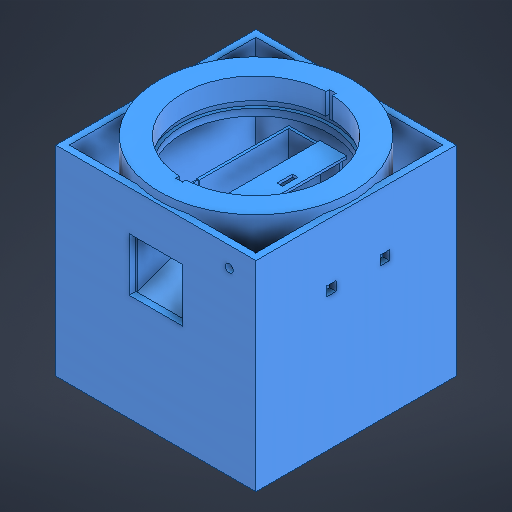
# Autodesk Inventor part: Box na elektrotechniku oprava
Saved by Autodesk Inventor 2026.2 (Build 302298000, 298)
## iProperties
Created: 2025-09-11
Part Number: Box na elektrotechniku oprava
Material: Všeobecné
Document SubType Name: Modeling
Designer: cerna
Density: 1 g/cm^3
Appearance: Světle modrá
Author: cerna
Autodesk Inventor part; units mm, degrees
sketch "Náčrt1" plane through (0, 0, 0) normal (0, 0, 1) x (1, 0, 0)
  line L0 (0, 105) -> (0, -105) projected
  line L1 (-105, 0) -> (105, 0) projected
  line L2 (-75, 75) -> (75, 75)
  line L3 (75, 75) -> (75, -75)
  line L4 (75, -75) -> (-75, -75)
  line L5 (-75, -75) -> (-75, 75)
  point P0 (0, 0)
  dimension "d0" = 150
  dimension "d1" = 150
  constraints: 8 end point, 2 parallel, 1 horizontal, 1 perpendicular, 2 other
  measures "d0" distance of L3.end L4.end
  measures "d1" distance of L2.end L3.end
extrude "Vysunutí1" add sketch "Náčrt1" along normal blind 150
sketch "Náčrt2" plane through (-75, 75, 0) normal (0, 1, 0) x (1, 0, 0)
  line L0 (0, 0) -> (0, -150) projected
  line L1 (150, 0) -> (0, 0) projected
  line L2 (5, -145) -> (145, -145)
  line L3 (145, -145) -> (145, -5)
  line L4 (145, -5) -> (5, -5)
  line L5 (5, -5) -> (5, -145)
  point P0 (75, 0)
  dimension "d4" = 140
  dimension "d5" = 140
  dimension "d6" = 5
  dimension "d7" = 5
  constraints: 8 end point, 2 parallel, 1 horizontal, 1 perpendicular
  measures "d4" distance of L4.end L3.end
  measures "d5" distance of L3.end L2.end
  measures "d6" distance between parallel lines of L1 L4
  measures "d7" distance between parallel lines of L0 L5
extrude "Vysunutí2" cut sketch "Náčrt2" against normal blind 140
sketch "Náčrt3" plane through (0, 0, 150) normal (0, 0, 1) x (1, 0, 0)
  line L0 (-20, 45) -> (20, 45)
  line L1 (20, 45) -> (20, 5)
  line L2 (20, 5) -> (-20, 5)
  line L3 (-20, 5) -> (-20, 45)
  line L4 (0, 105) -> (0, -105) projected
  line L5 (-105, 0) -> (105, 0) projected
  line L6 (-75, -75) -> (75, -75) projected
  circle A0 centre (55, 60) radius 3
  line L7 (75, -75) -> (75, 75) projected
  line L8 (75, 75) -> (-75, 75) projected
  point P0 (0, 0)
  dimension "d10" = 40
  dimension "d11" = 40
  dimension "d12" = 80
  dimension "d13" = 6
  dimension "d14" = 20
  dimension "d15" = 15
  constraints: 8 end point, 2 parallel, 1 centre point, 1 horizontal, 1 perpendicular, 1 other
  measures "d10" distance of L1.end L2.end
  measures "d11" distance of L0.end L1.end
  measures "d12" distance between parallel lines of L6 L2
  measures "d13" diameter of A0
  measures "d14" distance from line of L7 A0.centre
  measures "d15" distance from line of L8 A0.centre
extrude "Vysunutí3" cut sketch "Náčrt3" against normal blind 10 contours L0 L4 L2 L3 | L0 L1 L2 L4 | A0
sketch "Náčrt4" plane through (-70, 75, 5) normal (0, 0, 1) x (1, 0, 0)
  line L0 (70, -120) -> (82, -120)
  line L1 (82, -120) -> (82, -110)
  line L2 (82, -110) -> (70, -110)
  line L3 (70, -110) -> (70, -120)
  line L4 (-5, -150) -> (145, -150) projected
  line L5 (145, -150) -> (145, 0) projected
  point P0 (70, -75)
  point P1 (70, -115)
  dimension "d18" = 12
  dimension "d19" = 10
  dimension "d20" = 30
  dimension "d21" = 75
  constraints: 8 end point, 2 parallel, 1 horizontal, 1 midpoint, 1 perpendicular
  measures "d18" distance of L2.end L1.end
  measures "d19" distance of L1.end L0.end
  measures "d20" distance between parallel lines of L4 L0
  measures "d21" distance from line of L5 point (70, -115)
extrude "Vysunutí4" cut sketch "Náčrt4" against normal blind 10
sketch "Náčrt5" plane through (75, -75, 0) normal (1, 0, 0) x (0, 0, -1)
  line L0 (0, 0) -> (0, 150) projected
  line L1 (0, 0) -> (-150, 0) projected
  line L2 (-97, 107) -> (-90, 107)
  line L3 (-90, 107) -> (-90, 100)
  line L4 (-90, 100) -> (-97, 100)
  line L5 (-97, 100) -> (-97, 107)
  line L6 (-57, 107) -> (-50, 107)
  line L7 (-50, 107) -> (-50, 100)
  line L8 (-50, 100) -> (-57, 100)
  line L9 (-57, 100) -> (-57, 107)
  point P0 (0, 75)
  point P1 (-75, 0)
  dimension "d24" = 7
  dimension "d25" = 7
  dimension "d26" = 90
  dimension "d27" = 100
  dimension "d184" = 7
  dimension "d185" = 7
  dimension "d186" = 100
  dimension "d187" = 50
  constraints: 16 end point, 4 parallel, 2 horizontal, 2 perpendicular, 1 midpoint
  measures "d24" distance of L3.end L4.end
  measures "d25" distance of L2.end L3.end
  measures "d26" distance between parallel lines of L0 L3
  measures "d27" distance from line of point (-75, 0) L4
  measures "d184" distance of L6.end L7.end
  measures "d185" distance of L7.end L8.end
  measures "d186" distance between parallel lines of L1 L8
  measures "d187" distance between parallel lines of L0 L7
extrude "Vysunutí5" cut sketch "Náčrt5" against normal blind 10
ref_plane "Pracovní rovina3" through (0, 75, 0) normal (0, 1, 0) x (-1, 0, 0)
sketch "Náčrt8" plane through (0, 75, 0) normal (0, 1, 0) x (-1, 0, 0)
  line L0 (70, 145) -> (70, 5) projected
  line L1 (-70, 145) -> (70, 145) projected
  line L2 (70, 5) -> (-70, 5) projected
  line L3 (0, 5) -> (0, 0) projected
  circle A0 centre (0, 75) radius 72.5
  point P0 (70, 75)
  point P1 (70, 75)
  dimension "d132" = 70
  dimension "d133" = 70
  dimension "d134" = 145
  constraints: 2 midpoint, 1 centre point, 1 coincident
  measures "d132" distance from line of point (0, 75) L2
  measures "d133" distance of point (70, 75) point (0, 75)
  measures "d134" diameter of A0
extrude "Vysunutí6" add sketch "Náčrt8" against normal blind 20 contours A0 L0 | L0 A0 L2 L1 | L1 A0 | A0 L3 L2 | L2 L3 A0
sketch "Náčrt10" plane through (0, 75, 0) normal (0, 1, 0) x (1, 0, 0)
  line L0 (-75, 0) -> (-75, -150) projected
  line L1 (75, 0) -> (-75, 0) projected
  point P0 (0, 0)
  point P1 (0, -75)
  point P2 (-75, -75)
  point P3 (0, 0)
  dimension "d38" = 75
  dimension "d39" = 75
  constraints: 2 midpoint
  measures "d38" distance of point (-75, -75) point (0, -75)
  measures "d39" distance of point (0, 0) point (0, -75)
hole "Díra1" at (0, 75, 75) direction (0, -1, 0) diameter 110 depth 50
sketch "Náčrt11" plane through (0, 0, 0) normal (1, 0, 0) x (0, 1, 0)
  line L0 (5, 150) -> (5, 145) projected
  line L1 (75, 145) -> (-65, 145) projected
  line L2 (45, 150) -> (45, 145) projected
  line L3 (55, 140) -> (55, 75) projected
  line L4 (55, 130) -> (75, 130) projected
  line L5 (45, 145) -> (55, 130)
  line L6 (55, 99) -> (23, 99)
  line L7 (23, 99) -> (5, 145)
  line L8 (23, 99) -> (23, 42)
  line L9 (55, 99) -> (55, 130)
  line L10 (2.8523, 145) -> (20.8523, 99)
  line L11 (20.8523, 99) -> (23, 99)
  line L12 (47.4037, 145) -> (55, 133.6056)
  line L13 (2.8523, 145) -> (5, 145)
  line L14 (45, 145) -> (47.4037, 145)
  line L15 (55, 130) -> (55, 133.6056)
  point P0 (0, 0)
  dimension "d51" = 32
  dimension "d52" = 46
  dimension "d53" = 57
  dimension "d54" = 2
  dimension "d55" = 2
  constraints: 22 end point, 3 horizontal, 2 collinear, 2 parallel, 2 point on line, 1 perpendicular, 3 other
  measures "d51" distance of L6.start L6.end
  measures "d53" distance of L6.end L8.end
  measures "d54" distance between parallel lines of L7 L10
  measures "d55" distance between parallel lines of L12 L5
extrude "Vysunutí8" add sketch "Náčrt11" along normal mid plane 40 contours L12 L3 L5 L1 | L7 L11 L10 L1
sketch "Náčrt14" plane through (-20, 0, 0) normal (-1, 0, 0) x (0, 0, 1)
  line L0 (99, 20.8523) -> (99, 23) projected
  line L1 (99, 23) -> (99, 55)
  line L2 (130, 55) -> (20, 55) projected
  line L3 (145, 45) -> (130, 55) projected
  line L4 (130, 55) -> (145, 45)
  line L5 (145, 5) -> (145, 45) projected
  line L6 (145, 45) -> (145, 5)
  line L7 (99, 23) -> (145, 5) projected
  line L8 (145, 5) -> (99, 23)
  point P0 (0, 0)
  constraints: 8 end point, 3 collinear, 1 point on line, 1 vertical
extrude "Vysunutí9" add sketch "Náčrt14" against normal blind 1
sketch "Náčrt15" plane through (20, 0, 0) normal (1, 0, 0) x (0, 0, -1)
  line L0 (-145, 75) -> (-145, -65) projected
  line L1 (-99, 23) -> (-145, 5) projected
  line L2 (-145, 5) -> (-99, 23)
  line L3 (-99, 23) -> (-99, 55) projected
  line L4 (-99, 23) -> (-99, 55)
  line L5 (-99, 55) -> (-130, 55)
  line L6 (-145, 45) -> (-130, 55) projected
  line L7 (-130, 55) -> (-145, 45)
  line L8 (-145, 45) -> (-145, 5)
  point P0 (0, 0)
  constraints: 10 end point, 3 collinear, 2 perpendicular, 1 midpoint
extrude "Vysunutí10" add sketch "Náčrt15" against normal blind 1
ref_plane "Pracovní rovina8" through (19.5, 0, 0) normal (1, 0, 0) x (0, 0, -1)
sketch "Náčrt16" plane through (19.5, 0, 0) normal (1, 0, 0) x (0, 0, -1)
  line L0 (-99, 55) -> (-99, 23) projected
  line L1 (-99, 20.8523) -> (-145, 2.8523) projected
  line L2 (-126.614, 55) -> (-99, 55) projected
  line L3 (-99, 20.8523) -> (-32, 20.8523)
  line L4 (-32, 20.8523) -> (-32, 55)
  line L5 (-32, 20.8523) -> (-30, 20.8523)
  line L6 (-30, 20.8523) -> (-30, 55)
  line L7 (-30, 55) -> (-32, 55)
  point P0 (0, 0)
  point P1 (-130, 55)
  dimension "d69" = 67
  dimension "d70" = 2
  constraints: 10 end point, 3 perpendicular, 2 horizontal
  measures "d69" distance of L1.start L3.end
  measures "d70" distance of L3.end L5.end
extrude "Vysunutí11" add sketch "Náčrt16" against normal blind 40
sketch "Náčrt17" plane through (19.5, 20.8523, 32) normal (0, 0, 1) x (1, 0, 0)
  line L0 (-40, 34.1477) -> (-40, 0) projected
  line L1 (0, 0) -> (-40, 0) projected
  line L2 (0, 34.1477) -> (-40, 34.1477) projected
  line L3 (-40, 0) -> (-40, 34.1477)
  line L4 (-40, 34.1477) -> (-38, 34.1477)
  line L5 (-38, 34.1477) -> (-38, 0)
  point P0 (-19.5, -20.8523)
  dimension "d73" = 2
  constraints: 6 end point, 2 point on line, 1 collinear, 1 perpendicular
  measures "d73" distance of L0.start L4.end
extrude "Vysunutí12" add sketch "Náčrt17" along normal blind 67
ref_plane "Pracovní rovina10" through (19, 23, 99) normal (0, 0, -1) x (-1, 0, 0)
sketch "Náčrt20" plane through (19, 23, 99) normal (0, 0, -1) x (-1, 0, 0)
  line L0 (0, -18) -> (0, 22) projected
  line L1 (0, -18) -> (0, 0) projected
  line L2 (0, 0) -> (37.5, 0) projected
  line L3 (37.5, 0) -> (38, 0) projected
  line L4 (38, 0) -> (38, -18) projected
  line L5 (38, -18) -> (0, -18) projected
  line L6 (38, 0) -> (1.4186, 0)
  line L7 (38, 32) -> (19, 32) projected
  line L8 (19, 32) -> (0, 32) projected
  line L9 (1.4186, 0) -> (1.4186, 32)
  line L10 (1.4186, 0) -> (1.4186, -18)
  line L11 (1.4186, -18) -> (-0.5814, -18)
  line L12 (-0.5814, -18) -> (-0.5814, 32)
  line L13 (-0.5814, 32) -> (1.4186, 32)
  line L14 (38, 0) -> (16, 0)
  line L15 (16, 0) -> (16, 32)
  line L16 (16, 32) -> (14, 32)
  line L17 (14, 32) -> (14, -18)
  line L18 (14, -18) -> (16, -18)
  line L19 (-1, -18) -> (39, -18) projected
  line L20 (16, 0) -> (16, -18)
  line L21 (-0.5814, 32) -> (-4.5814, 32)
  line L22 (-4.5814, 32) -> (-4.5814, -18)
  line L23 (-4.5814, -18) -> (-6.5814, -18)
  line L24 (-6.5814, -18) -> (-6.5814, 32)
  line L25 (-6.5814, 32) -> (-4.5814, 32)
  line L26 (-6.5814, -18) -> (-6.5814, -20.025)
  line L27 (-6.5814, -20.025) -> (-4.5814, -20.025)
  line L28 (-4.5814, -20.025) -> (-4.5814, -18)
  line L29 (-0.5814, -18) -> (-0.5814, -22)
  line L30 (-0.5814, -22) -> (1.4186, -22)
  line L31 (1.4186, -22) -> (1.4186, -18)
  line L32 (-6.5814, -20.025) -> (-6.5814, -22)
  line L33 (-6.5814, -22) -> (-4.5814, -22)
  line L34 (-4.5814, -22) -> (-4.5814, -20.025)
  line L35 (14, -18) -> (14, -22)
  line L36 (14, -22) -> (16, -22)
  line L37 (16, -22) -> (16, -18)
  point P0 (19, -23)
  point P1 (0, 32)
  point P2 (-5.5814, -18)
  point P3 (-5.5814, 32)
  dimension "d83" = 2
  dimension "d84" = 22
  dimension "d85" = 2
  dimension "d86" = 4
  dimension "d87" = 2
  dimension "d94" = 50
  dimension "d95" = 50
  dimension "d96" = 4
  constraints: 58 end point, 18 point on line, 14 perpendicular, 2 midpoint, 2 parallel, 2 vertical, 2 other
  measures "d83" distance of L10.end L11.end
  measures "d84" distance of L3.end L14.end
  measures "d85" distance of L15.end L16.end
  measures "d86" distance of L12.end L21.end
  measures "d87" distance of L22.end L23.end
  measures "d94" distance of point (-5.581, -18) point (-5.581, 32)
  measures "d95" distance of L23.end L24.end
  measures "d96" distance of L11.end L29.end
extrude "Vysunutí14" add sketch "Náčrt20" along normal blind 67 contours L17 L2 L20 L5 | L5 L37 L36 L35 | L17 L8 L15 L2
ref_plane "Pracovní rovina11" through (-75, 60, 0) normal (0, 1, 0) x (1, 0, 0)
sketch "Náčrt26" plane through (-75, 60, 0) normal (0, 1, 0) x (1, 0, 0)
  circle A0 centre (75, -75) radius 55 projected
  line L0 (75, -5) -> (75, 0) projected
  arc A1 (56.1254, -5) -> (5, -56.1254) centre (75, -75) ccw projected
  circle A2 centre (75, -75) radius 57.5
  dimension "d136" = 115
  constraints: 2 coincident, 1 centre point
  measures "d136" diameter of A2
hole "Díra3" at (0, 60, 75) direction (0, 1, 0) diameter 115 depth 5
sketch "Náčrt28" plane through (5, 23, 99) normal (1, 0, 0) x (0, 0, -1)
  line L0 (0, 32) -> (67, 32) projected
  line L1 (0, 32) -> (2, 32)
  line L2 (2, 32) -> (2, -22)
  line L3 (2, -22) -> (0, -22)
  line L4 (0, -22) -> (0, 32)
  point P0 (99, -23)
  point P1 (2, 32)
  point P2 (50, 32)
  dimension "d157" = 2
  dimension "d158" = 54
  constraints: 8 end point, 2 parallel, 1 horizontal, 1 perpendicular
  measures "d157" distance of L2.end L3.end
  measures "d158" distance of L1.end L2.end
extrude "Vysunutí20" add sketch "Náčrt28" along normal blind 15
sketch "Náčrt27" plane through (0, 65, 75) normal (0, -1, 0) x (1, 0, 0)
  circle A0 centre (0, 0) radius 55 projected
  line L0 (-2.5, -57.5) -> (2.5, -57.5)
  line L1 (2.5, -57.5) -> (2.5, -50)
  line L2 (2.5, -50) -> (-2.5, -50)
  line L3 (-2.5, -50) -> (-2.5, -57.5)
  line L4 (0, 105) -> (0, -105) projected
  line L5 (75, -75) -> (-75, -75) projected
  line L6 (2.5, 50) -> (2.5, 57.5)
  line L7 (2.5, 57.5) -> (-2.5, 57.5)
  line L8 (-2.5, 57.5) -> (-2.5, 50)
  line L9 (-2.5, 50) -> (2.5, 50)
  circle A1 centre (0, 0) radius 57.5 projected
  point P0 (0, -75)
  point P1 (52.6504, -23.1124)
  point P2 (-52.6504, -23.1124)
  dimension "d146" = 5
  dimension "d148" = 25
  dimension "d155" = 360
  constraints: 16 end point, 2 parallel, 1 horizontal, 1 perpendicular, 1 tangent, 19 other
  measures "d146" distance between parallel lines of L1 L3
  measures "d148" distance between parallel lines of L5 L2
extrude "Vysunutí19" cut sketch "Náčrt27" along normal blind 3 and the other way blind 10 contours L6 L9 L4 A0 | A0 L4 A1 L6 | L1 A1 L4 A0 | A0 L4 L2 L1 | L4 L9 L8 A0 | A0 L8 A1 L4 | A1 L7 L6 | L4 A1 L3 A0 | A0 L3 L2 L4 | L1 L0 A1 | A1 L8 L7 | L0 L3 A1
sketch "Náčrt30" plane through (-75, 75, 0) normal (0, 1, 0) x (1, 0, 0)
  arc A0 (56.1254, -5) -> (5, -56.1254) centre (75, -75) ccw projected
  arc A1 (72.5, -20.0568) -> (72.5, -129.9432) centre (75, -75) ccw projected
  circle A2 centre (75, -75) radius 72.5
  circle A3 centre (75, -75) radius 55
  point P0 (75, 0)
  point P1 (72.5, -129.9432)
  point P2 (5, -56.1254)
  point P3 (56.1254, -5)
  constraints: 2 centre point, 2 coincident, 2 concentric
extrude "Vysunutí22" add sketch "Náčrt30" along normal blind 6
sketch "Náčrt31" plane through (0, 81, 75) normal (0, 1, 0) x (1, 0, 0)
  circle A0 centre (0, 0) radius 55 projected
  line L0 (-2.5, 54.9432) -> (-2.5, 57.5) projected
  line L1 (-2.5, 57.5) -> (2.5, 57.5) projected
  line L2 (2.5, 57.5) -> (2.5, 54.9432) projected
  line L3 (-2.5, -57.5) -> (-2.5, -54.9432) projected
  line L4 (2.5, -57.5) -> (-2.5, -57.5) projected
  line L5 (2.5, -54.9432) -> (2.5, -57.5) projected
  line L6 (-2.5, -57.5) -> (2.5, -57.5)
  line L7 (2.5, -57.5) -> (2.5, -53.9565)
  line L8 (2.5, -53.9565) -> (-2.5, -53.9565)
  line L9 (-2.5, -53.9565) -> (-2.5, -57.5)
  line L10 (2.5, 57.5) -> (-2.5, 57.5)
  line L11 (-2.5, 57.5) -> (-2.5, 54.0591)
  line L12 (-2.5, 54.0591) -> (2.5, 54.0591)
  line L13 (2.5, 54.0591) -> (2.5, 57.5)
  point P0 (0, 75)
  dimension "d166" = 3.5435
  dimension "d167" = 3.4409
  constraints: 16 end point, 4 parallel, 2 horizontal, 2 perpendicular, 1 point on line
  measures "d166" distance between parallel lines of L8 L4
  measures "d167" distance between parallel lines of L1 L12
extrude "Vysunutí23" cut sketch "Náčrt31" against normal blind 6 contours A0 L0 L1 L2 | L5 L4 L3 A0
sketch "Náčrt32" plane through (-19, 5, 145) normal (0, 0.9312, 0.3644) x (1, 0, 0)
  line L0 (22, 49.3964) -> (0.5, 49.3964) projected
  line L1 (0.5, 49.3964) -> (22, 49.3964)
  line L2 (22, 49.3964) -> (22, 47.3964)
  line L3 (22, 47.3964) -> (0.5, 47.3964)
  line L4 (0.5, 47.3964) -> (0.5, 49.3964)
  point P0 (19, 133.2082)
  point P1 (22, 49.3964)
  dimension "d171" = 2
  constraints: 8 end point, 2 parallel, 1 horizontal, 1 perpendicular
  measures "d171" distance of L1.end L2.end
extrude "Vysunutí24" cut sketch "Náčrt32" against normal blind 8
sketch "Náčrt33" plane through (3, 55, 99) normal (0, 1, 0) x (1, 0, 0)
  line L0 (0, 0) -> (17, 0) projected
  line L1 (0, 0) -> (16.5, 0)
  line L2 (16.5, 69) -> (0, 69)
  line L3 (0, 69) -> (0, 0)
  line L4 (16.5, 67) -> (2, 67) projected
  line L5 (16.5, 69) -> (-23.5, 69) projected
  line L6 (16.5, 69) -> (16.5, 67) projected
  line L7 (11.5, 25.25) -> (15.6, 25.25)
  line L8 (15.6, 25.25) -> (15.6, 36.75)
  line L9 (15.6, 36.75) -> (11.5, 36.75)
  line L10 (11.5, 36.75) -> (11.5, 25.25)
  line L11 (20, 0) -> (20, 69)
  line L12 (20, 69) -> (16.5, 69)
  line L13 (20, 0) -> (16.5, 0)
  line L14 (0, 0) -> (0, 67) projected
  line L15 (2, 35) -> (2, 35) projected
  line L16 (2, 31) -> (22.5208, 31)
  line L17 (2, 35) -> (2, 35)
  line L18 (0, 35) -> (0, 27)
  point P0 (-3, 99)
  point P1 (0, 51)
  dimension "d174" = 11.5
  dimension "d175" = 4.1
  dimension "d176" = 20
  dimension "d177" = 11.5
  constraints: 26 end point, 4 parallel, 3 perpendicular, 2 horizontal, 2 point on line, 1 collinear, 1 vertical, 1 other
  measures "d174" distance between parallel lines of L10 L3
  measures "d175" distance between parallel lines of L10 L8
  measures "d176" distance from line of point (0, 51) L11
  measures "d177" distance between parallel lines of L9 L7
extrude "Vysunutí25" add sketch "Náčrt33" along normal blind 2
sketch "Náčrt34" plane through (3, 1, 99) normal (-1, 0, 0) x (0, 0, 1)
  line L0 (0, 19.8523) -> (0, 0) projected
  line L1 (-67, 54) -> (-67, 19.8523) projected
  line L2 (0, 19.8523) -> (-67, 19.8523)
  line L3 (-67, 19.8523) -> (-67, 22)
  line L4 (-67, 22) -> (-67, 19.8523)
  line L5 (-2, 0) -> (-2, 54) projected
  line L6 (0, 54) -> (0, 22) projected
  line L7 (0, 22) -> (0, 19.8523)
  line L8 (46, 4) -> (0, 22) projected
  line L9 (0, 22) -> (-67, 27.9965)
  line L10 (-67, 19.8523) -> (-67, 0) projected
  line L11 (-67, 19.8523) -> (-67, 27.9965)
  point P0 (-99, -1)
  constraints: 12 end point, 2 collinear, 2 point on line, 1 horizontal
extrude "Vysunutí26" add sketch "Náčrt34" along normal blind 22
sketch "Náčrt35" plane through (3, 20.8523, 99) normal (-1, 0, 0) x (0, 0, 1)
  line L0 (0, 0) -> (0, -19.8523) projected
  line L1 (0, 0) -> (-2, 0)
  line L2 (-2, -19.8523) -> (-2, 34.1477) projected
  line L3 (-2, 0) -> (-2, 2.3389)
  line L4 (-2, 2.3389) -> (0, 2.1477)
  line L5 (0, 2.1477) -> (5.4885, 0)
  line L6 (46, -15.8523) -> (0, 2.1477) projected
  line L7 (0, 0) -> (5.4885, 0)
  point P0 (-99, -20.8523)
  constraints: 10 end point, 4 point on line, 1 horizontal, 1 perpendicular
extrude "Vysunutí27" add sketch "Náčrt35" along normal blind 22
